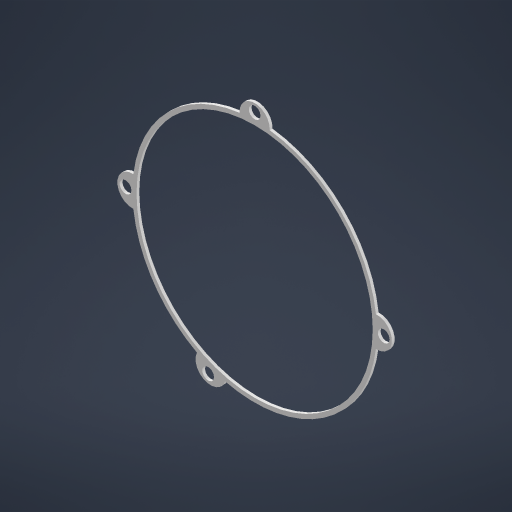
# Autodesk Inventor part: big_funny_washer
Saved by Autodesk Inventor 2024.2 (Build 282272000, 272)
## iProperties
Created: 2024-03-29
Part Number: big_funny_washer
Material: Generic
Document SubType Name: Modeling
Designer: warm
Density: 1 g/cm^3
Appearance: Default
Author: warm
Autodesk Inventor part; units mm, degrees
ref_plane "YZ Plane" through (0, 0, 0) normal (1, 0, 0) x (0, 1, 0)
ref_plane "XZ Plane" through (0, 0, 0) normal (0, 1, 0) x (-1, 0, 0)
ref_plane "XY Plane" through (0, 0, 0) normal (0, 0, 1) x (1, 0, 0)
sketch "Sketch1" plane through (0, 0, 0) normal (0, 0, 1) x (1, 0, 0)
  circle A0 centre (43.1089, 0) radius 44.45 projected
  circle A1 centre (43.1089, 0) radius 42.95
  line L0 (43.1089, -44.45) -> (43.1089, 44.45)
  line L1 (43.1089, 44.45) -> (43.1089, 62.0895)
  line L2 (87.5589, 0) -> (-1.3411, 0)
  circle A2 centre (43.1089, 44.45) radius 5.5
  circle A3 centre (87.5589, 0) radius 5.5
  circle A4 centre (-1.3411, 0) radius 5.5
  circle A5 centre (27.1089, -41.4705) radius 5.5
  point P0 (0, 0)
  point P1 (48.5984, 44.1097)
  point P2 (37.6194, 44.1097)
  point P3 (-1.0008, 5.4895)
  point P4 (-1.0008, -5.4895)
  point P5 (87.2186, -5.4895)
  point P6 (87.2186, 5.4895)
  point P7 (43.1089, 0)
  point P8 (32.3529, -43.129)
  point P9 (22.1099, -39.1771)
  dimension "d0" = 1.5
  dimension "d1" = 0
  dimension "d2" = 88.9
  dimension "d3" = 44.45
  dimension "d4" = 88.9
  dimension "d5" = 0
  dimension "d6" = 44.45
  dimension "d7" = 11
  dimension "d8" = 11
  dimension "d10" = 11
  dimension "d27" = 11
  dimension "d29" = 44.45
  dimension "d30" = 16
  constraints: 6 end point, 5 centre point, 3 coincident, 1 midpoint, 1 perpendicular, 1 point on line, 1 vertical
  measures "d0" radial gap between concentric circles of A0 A1
  measures "d1" vertical distance of A0.centre L2.start
  measures "d2" distance of L2.start L2.end
  measures "d3" distance of A0.centre L2.start
  measures "d4" distance of L0.start L0.end
  measures "d5" distance from line of A0.centre L0
  measures "d6" distance of A0.centre L0.end
  measures "d7" diameter of A2
  measures "d8" diameter of A3
  measures "d10" diameter of A4
  measures "d27" diameter of A5
  measures "d29" distance of point (43.109, 0) A5.centre
  measures "d30" horizontal distance of L0.start A5.centre
extrude "Extrusion1" add sketch "Sketch1" along normal blind 1 contours L2 A1 A3 A0 | A0 A3 | A0 A3 A1 L2 | A3 A1 A2 A0 | A0 L0 A1 A3 | A2 A1 L0 A0 | A0 L1 A2 | A0 A5 A1 L0 | L0 A1 A2 A0 | A0 A2 L1 | A5 A0 | A0 A5 A1 | A2 A1 A4 A0 | A0 A4 A1 A5 | A4 A1 L2 A0 | A0 A4 | A0 L2 A1 A4
sketch "Sketch2" plane through (0, 0, 1) normal (0, 0, 1) x (1, 0, 0)
  circle A0 centre (43.1089, 46.9519) radius 2.15
  arc A1 (-1.0008, -5.4895) -> (48.5984, 44.1097) centre (43.1089, 0) ccw projected
  arc A2 (48.5984, 44.1097) -> (37.6194, 44.1097) centre (43.1089, 44.45) ccw projected
  circle A3 centre (43.1089, 0) radius 44.45
  circle A4 centre (90.0608, 0) radius 2.15
  circle A5 centre (-3.843, 0) radius 2.15
  arc A6 (87.2186, -5.4895) -> (87.2186, 5.4895) centre (87.5589, 0) ccw projected
  arc A7 (-1.0008, 5.4895) -> (-1.0008, -5.4895) centre (-1.3411, 0) ccw projected
  circle A8 centre (26.2083, -43.8047) radius 2.15
  arc A9 (22.1099, -39.1771) -> (32.3529, -43.129) centre (27.1089, -41.4705) ccw projected
  point P0 (0, 0)
  point P1 (25.1291, -46.6018)
  point P2 (25.1291, -46.6018)
  point P3 (-6.8411, 0)
  dimension "d13" = 4.3
  dimension "d14" = 2.5019
  dimension "d15" = 0
  dimension "d16" = 4.3
  dimension "d18" = 4.3
  dimension "d19" = 0
  dimension "d20" = 2.5019
  dimension "d23" = 0
  dimension "d24" = 2.5019
  dimension "d31" = 4.3
  dimension "d33" = 2.5019
  dimension "d35" = 2.9981
  dimension "d36" = 5.5
  constraints: 5 centre point, 4 point on circle, 1 coincident
  measures "d13" diameter of A0
  measures "d14" distance of A2.centre A0.centre
  measures "d15" horizontal distance of A2.centre A0.centre
  measures "d16" diameter of A4
  measures "d18" diameter of A5
  measures "d19" vertical distance of A7.centre A5.centre
  measures "d20" distance of A7.centre A5.centre
  measures "d23" vertical distance of A6.centre A4.centre
  measures "d24" distance of A6.centre A4.centre
  measures "d31" diameter of A8
  measures "d33" distance of A9.centre A8.centre
  measures "d35" distance of point (25.129, -46.602) A8.centre
  measures "d36" distance of point (-6.841, 0) A7.centre
extrude "Extrusion2" cut sketch "Sketch2" against normal through all contours A0 | A4 | A5 | A8
equation "\"d3\" = 0.5 * d2"
equation "\"d4\" = d2"
equation "\"d6\" = d3"
equation "\"d8\" = d7"
equation "\"d10\" = d7"
equation "\"d27\" = d28"
equation "\"d29\" = d3"
equation "\"d20\" = d14"
equation "\"d24\" = d22"
equation "\"d33\" = d20"
equation "\"d35\" = d36 - d20"
equation "\"d22\" = d20"
equation "\"d28\" = 11"
body "Solid1"
